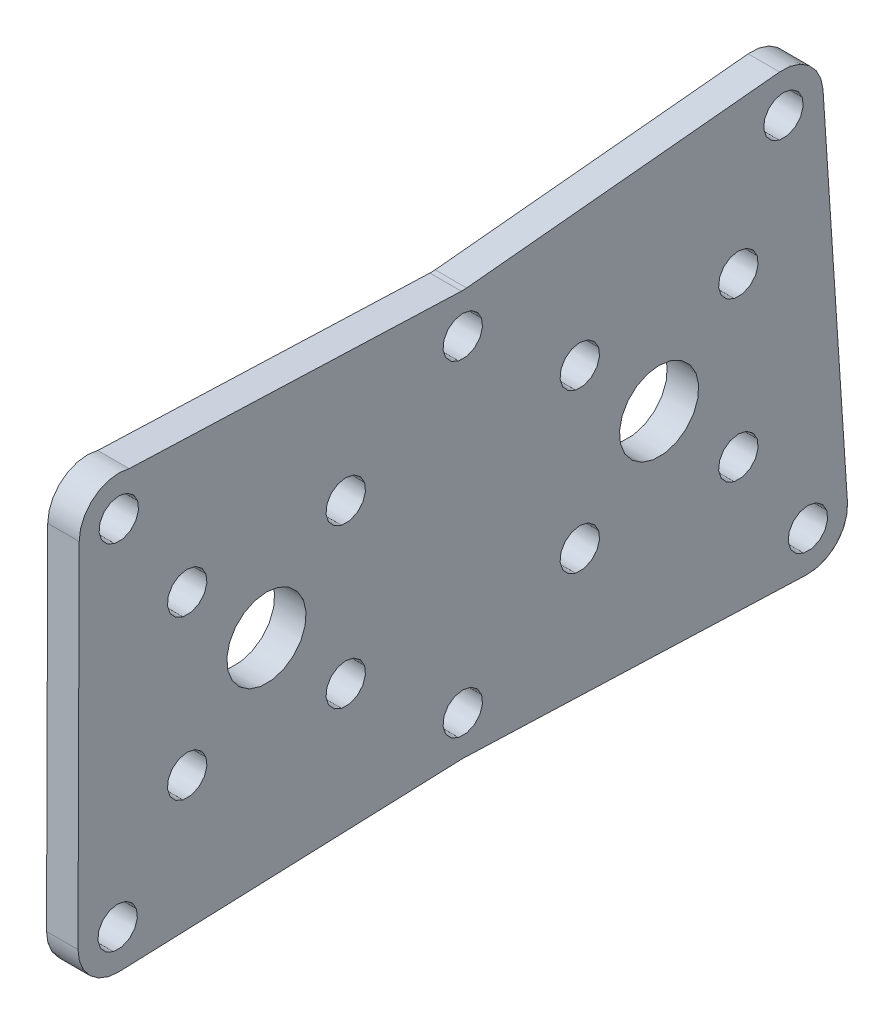
# Autodesk Inventor part: motorMountPlate2.0
Saved by Autodesk Inventor 2023 (Build 270158000, 158)
## iProperties
Created: 2022-09-08
Part Number: motorMountPlate2.0
Material: Generic
Document SubType Name: Modeling
Designer: deli
Density: 1 g/cm^3
Appearance: Default
Author: deli
Autodesk Inventor part; units mm, degrees
ref_plane "YZ Plane" through (0, 0, 0) normal (1, 0, 0) x (0, 1, 0)
ref_plane "XZ Plane" through (0, 0, 0) normal (0, 1, 0) x (-1, 0, 0)
ref_plane "XY Plane" through (0, 0, 0) normal (0, 0, 1) x (1, 0, 0)
sketch "Sketch1" plane through (0, 0, 0) normal (1, 0, 0) x (0, 1, 0)
  circle A0 centre (49.8613, -14.2667) radius 2 projected
  circle A1 centre (14.2614, -14.1478) radius 2 projected
  circle A2 centre (15.5588, -48.9729) radius 2 projected
  circle A3 centre (48.4639, -48.9729) radius 2 projected
  circle A4 centre (51.5846, -81.3294) radius 2 projected
  circle A5 centre (14.2614, -83.7981) radius 2 projected
  circle A6 centre (32.0114, -29.1644) radius 7 construction
  circle A7 centre (32.0114, -68.7814) radius 7 construction
  circle A8 centre (32.0114, -29.1644) radius 4
  circle A9 centre (32.0114, -68.7814) radius 4
  circle A10 centre (32.0114, -29.1644) radius 9.3137 construction
  circle A11 centre (32.0114, -68.7814) radius 9.3137 construction
  arc A12 (53.7203, -15.3194) -> (49.8747, -10.2668) centre (49.8613, -14.2667) ccw
  circle A13 centre (48.4639, -48.9729) radius 4 construction
  circle A14 centre (15.5588, -48.9729) radius 4 construction
  arc A15 (14.2747, -10.1478) -> (10.2642, -14.2973) centre (14.2614, -14.1478) ccw
  arc A16 (10.2642, -83.6485) -> (14.5254, -87.7893) centre (14.2614, -83.7981) ccw
  arc A17 (51.8486, -85.3207) -> (55.5656, -80.9408) centre (51.5846, -81.3294) ccw
  arc A18 (52.4667, -48.8234) -> (52.4829, -49.3616) centre (56.4639, -48.9729) ccw
  arc A19 (11.556, -49.1225) -> (11.556, -48.8234) centre (7.5588, -48.9729) ccw
  circle A20 centre (40.0114, -21.1644) radius 2
  circle A21 centre (40.0114, -37.1644) radius 2
  circle A22 centre (24.0114, -21.1644) radius 2
  circle A23 centre (24.0114, -37.1644) radius 2
  circle A24 centre (24.0114, -60.7814) radius 2
  circle A25 centre (24.0114, -76.7814) radius 2
  circle A26 centre (40.0114, -76.7814) radius 2
  circle A27 centre (40.0114, -60.7814) radius 2
  line L0 (40.0114, -21.1644) -> (40.0114, -37.1644) construction
  line L1 (40.0114, -37.1644) -> (24.0114, -37.1644) construction
  line L2 (24.0114, -37.1644) -> (24.0114, -21.1644) construction
  line L3 (24.0114, -21.1644) -> (40.0114, -21.1644) construction
  line L4 (40.0114, -60.7814) -> (40.0114, -76.7814) construction
  line L5 (40.0114, -76.7814) -> (24.0114, -76.7814) construction
  line L6 (24.0114, -76.7814) -> (24.0114, -60.7814) construction
  line L7 (40.0114, -60.7814) -> (24.0114, -60.7814) construction
  line L8 (53.7203, -15.3194) -> (52.4667, -48.8234)
  line L9 (52.4829, -49.3616) -> (55.5656, -80.9408)
  line L10 (51.8486, -85.3207) -> (14.5254, -87.7893)
  line L11 (10.2642, -83.6485) -> (11.556, -49.1225)
  line L12 (11.556, -48.8234) -> (10.2642, -14.2973)
  line L13 (14.2747, -10.1478) -> (49.8747, -10.2668)
  point P0 (0, 0)
  dimension "d0" = 8
  dimension "d1" = 8
  dimension "d2" = 8
  dimension "d3" = 8
  dimension "d4" = 8
  dimension "d5" = 8
  dimension "d6" = 8
  dimension "d7" = 0
  dimension "d8" = 8
  dimension "d9" = 0
  dimension "d10" = 4
  dimension "d11" = 4
  dimension "d12" = 4
  dimension "d13" = 4
  dimension "d14" = 4
  dimension "d15" = 4
  dimension "d16" = 4
  dimension "d17" = 4
  dimension "d18" = 8
  dimension "d19" = 8
  dimension "d20" = 16
  dimension "d21" = 16
  dimension "d22" = 16
  dimension "d23" = 16
  constraints: 28 end point, 21 tangent, 20 centre point, 12 point on circle, 10 coincident, 3 perpendicular, 2 vertical, 1 collinear, 1 parallel
  measures "d0" diameter of A12
  measures "d1" diameter of A18
  measures "d2" diameter of A15
  measures "d3" diameter of A14
  measures "d4" diameter of A19
  measures "d5" diameter of A16
  measures "d6" diameter of A17
  measures "d7" vertical distance of A18.centre A3.centre
  measures "d8" diameter of A13
  measures "d9" vertical distance of A14.centre A19.centre
  measures "d10" diameter of A22
  measures "d11" diameter of A23
  measures "d12" diameter of A21
  measures "d13" diameter of A20
  measures "d14" diameter of A27
  measures "d15" diameter of A24
  measures "d16" diameter of A25
  measures "d17" diameter of A26
  measures "d18" diameter of A8
  measures "d19" diameter of A9
  measures "d20" distance of L0.start L0.end
  measures "d21" distance of L2.end L0.start
  measures "d22" distance of L4.start L6.end
  measures "d23" distance of L4.start L4.end
extrude "Extrusion1" add sketch "Sketch1" along normal blind 3.175
equation "\"d1\" = d0"
equation "\"d2\" = d0"
equation "\"d3\" = d0"
equation "\"d4\" = d0"
equation "\"d5\" = d0"
equation "\"d6\" = d0"
equation "\"d8\" = d0"
equation "\"d11\" = d10"
equation "\"d12\" = d10"
equation "\"d13\" = d10"
equation "\"d14\" = d10"
equation "\"d15\" = d10"
equation "\"d16\" = d10"
equation "\"d17\" = d10"
equation "\"d18\" = d0"
equation "\"d19\" = d0"
equation "\"d21\" = d20"
equation "\"d22\" = d20"
equation "\"d23\" = d20"
body "Solid1"
